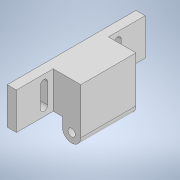
# Autodesk Inventor part: Hinge - V2
Saved by Autodesk Inventor 2022 (Build 260153000, 153)
## iProperties
Created: 2022-06-13
Part Number: Hinge - V2
Material: Generic
Document SubType Name: Modeling
Designer: Caleb
Density: 1 g/cm^3
Appearance: Default
Author: Caleb
Autodesk Inventor part; units mm, degrees
ref_plane "YZ Plane" through (0, 0, 0) normal (1, 0, 0) x (0, 1, 0)
ref_plane "XZ Plane" through (0, 0, 0) normal (0, 1, 0) x (-1, 0, 0)
ref_plane "XY Plane" through (0, 0, 0) normal (0, 0, 1) x (1, 0, 0)
sketch "Sketch1" plane through (0, 0, 0) normal (0, 1, 0) x (-1, 0, 0)
  line L0 (-6.35, -15.875) -> (6.35, -15.875)
  line L1 (6.35, -15.875) -> (6.35, 15.875)
  line L2 (6.35, 15.875) -> (-6.35, 15.875)
  line L3 (-6.35, 15.875) -> (-6.35, -15.875)
  line L4 (-6.35, -15.875) -> (6.35, 15.875) construction
  line L5 (6.35, -15.875) -> (-6.35, 15.875) construction
  point P0 (0, 0)
  dimension "d0" = 12.7
  dimension "d1" = 31.75
  constraints: 12 end point, 2 midpoint, 2 parallel, 1 horizontal, 1 perpendicular
  measures "d0" distance of L2.end L1.end
  measures "d1" distance of L1.end L0.end
extrude "Extrusion1" add sketch "Sketch1" along normal blind 19.05
sketch "Sketch2" plane through (0, 19.05, 0) normal (0, 1, 0) x (1, 0, 0)
  line L0 (6.35, -15.875) -> (6.35, 15.875) projected
  line L1 (6.35, 15.875) -> (-3.175, 15.875)
  line L2 (-3.175, 15.875) -> (-3.175, 3.175)
  line L3 (-3.175, 3.175) -> (6.35, 3.175)
  line L4 (6.35, 3.175) -> (6.35, 15.875)
  line L5 (-6.35, 15.875) -> (-6.35, -15.875) projected
  point P0 (0, 0)
  dimension "d4" = 12.7
  dimension "d5" = 3.175
  constraints: 8 end point, 2 parallel, 1 horizontal, 1 perpendicular
  measures "d4" distance of L1.end L2.end
  measures "d5" distance between parallel lines of L5 L2
extrude "Extrusion2" cut sketch "Sketch2" against normal through all
sketch "Sketch3" plane through (-6.35, 0, 15.875) normal (0, 0, 1) x (1, 0, 0)
  line L0 (0, 0) -> (6.35, 0)
  line L1 (6.35, 0) -> (6.35, 6.35)
  line L2 (6.35, 6.35) -> (0, 6.35)
  line L3 (0, 6.35) -> (0, 0)
  point P0 (6.35, 0)
  dimension "d8" = 6.35
  dimension "d9" = 6.35
  constraints: 8 end point, 2 parallel, 1 horizontal, 1 perpendicular
  measures "d8" distance of L2.end L1.end
  measures "d9" distance of L1.end L0.end
extrude "Extrusion3" cut sketch "Sketch3" against normal through all
sketch "Sketch4" plane through (-6.35, 19.05, 15.875) normal (0, 0, 1) x (1, 0, 0)
  line L0 (0, -12.7) -> (0, 0) projected
  line L1 (3.175, 0) -> (3.175, -12.7) projected
  line L2 (0, -12.7) -> (3.175, -12.7)
  line L3 (3.175, -12.7) -> (3.175, 0)
  line L4 (3.175, 0) -> (0, 0)
  line L5 (0, 0) -> (0, -12.7)
  point P0 (6.35, -19.05)
  constraints: 8 end point, 2 parallel, 1 horizontal, 1 perpendicular
extrude "Extrusion4" add sketch "Sketch4" along normal blind 12.7
sketch "Sketch6" plane through (6.35, 0, 15.875) normal (0, 0, 1) x (1, 0, 0)
  line L0 (-6.35, 0) -> (0, 0) projected
  line L1 (0, 0) -> (0, 19.05) projected
  point P0 (-3.175, 3.175)
  point P1 (-3.175, 0)
  dimension "d18" = 3.175
  dimension "d19" = 3.175
  measures "d18" distance from line of L0 point (-3.175, 3.175)
  measures "d19" distance from line of L1 point (-3.175, 3.175)
hole "Hole1" at (3.175, 3.175, 15.875) direction (0, 0, -1) diameter 2.54 end through all
sketch "Sketch7" plane through (-3.175, 6.35, 15.875) normal (1, 0, 0) x (0, 0, -1)
  line L0 (-3.175, 2.8575) -> (-3.175, 9.8425) construction
  line L1 (-4.445, 2.8575) -> (-4.445, 9.8425)
  line L2 (-1.905, 9.8425) -> (-1.905, 2.8575)
  arc A0 (-4.445, 2.8575) -> (-1.905, 2.8575) centre (-3.175, 2.8575) ccw
  arc A1 (-1.905, 9.8425) -> (-4.445, 9.8425) centre (-3.175, 9.8425) ccw
  line L3 (-12.7, 0) -> (-12.7, 12.7) projected
  line L4 (0, 0) -> (-12.7, 0) projected
  line L5 (22.225, 2.8575) -> (22.225, 9.8425) construction
  line L6 (23.495, 2.8575) -> (23.495, 9.8425)
  line L7 (20.955, 9.8425) -> (20.955, 2.8575)
  arc A2 (20.955, 2.8575) -> (23.495, 2.8575) centre (22.225, 2.8575) ccw
  arc A3 (23.495, 9.8425) -> (20.955, 9.8425) centre (22.225, 9.8425) ccw
  line L8 (19.05, 0) -> (31.75, 0) projected
  line L9 (31.75, 12.7) -> (31.75, 0) projected
  point P0 (15.875, -6.35)
  point P1 (-3.175, 6.35)
  point P2 (22.225, 6.35)
  dimension "d27" = 6.985
  dimension "d28" = 9.525
  dimension "d29" = 6.35
  dimension "d30" = 2.54
  dimension "d31" = 2.54
  dimension "d32" = 6.35
  dimension "d33" = 6.985
  dimension "d34" = 9.525
  constraints: 16 end point, 8 point on circle, 8 tangent, 4 centre point, 2 midpoint, 2 parallel, 2 vertical
  measures "d27" distance of L0.start L0.end
  measures "d28" distance from line of L3 point (-3.175, 6.35)
  measures "d29" distance from line of L4 point (-3.175, 6.35)
  measures "d30" distance between parallel lines of L1 L2
  measures "d31" distance between parallel lines of L7 L6
  measures "d32" distance from line of L8 point (22.225, 6.35)
  measures "d33" distance of L5.end L5.start
  measures "d34" distance from line of L9 point (22.225, 6.35)
extrude "Extrusion6" cut sketch "Sketch7" against normal through all
sketch "Sketch8" plane through (6.35, 0, 15.875) normal (0, 0, 1) x (1, 0, 0)
  circle A0 centre (-3.175, 3.175) radius 1.27 projected
  line L0 (-6.35, 0) -> (-6.35, 6.35) projected
  line L1 (0, 0) -> (0, 19.05) projected
  arc A1 (-6.35, 3.175) -> (0, 3.175) centre (-3.175, 3.175) ccw
  line L2 (-6.35, 0) -> (0, 0) projected
  point P0 (-3.175, 0)
  constraints: 2 point on circle, 1 centre point, 1 coincident, 1 midpoint, 1 point on line
extrude "Extrusion7" cut sketch "Sketch8" against normal through all contours A1 L1 L2 | L0 A1 L2
equation "\"d19\" = d18"
equation "\"d31\" = d30"
equation "\"d32\" = d29"
equation "\"d33\" = d27"
equation "\"d34\" = d28"
body "Solid1"
